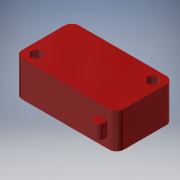
# Autodesk Inventor part: microswitch
Saved by Autodesk Inventor 2019 (Build 230136000, 136)
## iProperties
Created: 2021-01-21
Part Number: microswitch
Material: PET Plastic
Document SubType Name: Modeling
Designer: Juan M. Casillas
Density: 1.541 g/cm^3
Appearance: Smooth - Red
Author: Juan M. Casillas
Autodesk Inventor part; units mm, degrees
ref_plane "YZ Plane" through (0, 0, 0) normal (1, 0, 0) x (0, 1, 0)
ref_plane "XZ Plane" through (0, 0, 0) normal (0, 1, 0) x (-1, 0, 0)
ref_plane "XY Plane" through (0, 0, 0) normal (0, 0, 1) x (1, 0, 0)
sketch "Sketch1" plane through (0, 0, 0) normal (0, 1, 0) x (-1, 0, 0)
  line L0 (12, 7.85) -> (-12, 7.85)
  line L1 (-14, 5.85) -> (-14, -5.85)
  line L2 (-12, -7.85) -> (12, -7.85)
  line L3 (14, -5.85) -> (14, 5.85)
  line L4 (14, 7.85) -> (-14, -7.85) construction
  line L5 (-14, 7.85) -> (14, -7.85) construction
  arc A0 (14, 5.85) -> (12, 7.85) centre (12, 5.85) ccw
  arc A1 (12, -7.85) -> (14, -5.85) centre (12, -5.85) ccw
  arc A2 (-14, -5.85) -> (-12, -7.85) centre (-12, -5.85) ccw
  arc A3 (-12, 7.85) -> (-14, 5.85) centre (-12, 5.85) ccw
  line L6 (12.5, 8.7909) -> (12.5, -11.3064) construction
  line L7 (15.2914, 6.35) -> (1.3637, 6.35) construction
  circle A4 centre (11, 4.85) radius 1.5
  line L8 (14, 0) -> (-14, 0) construction
  line L9 (0, 7.85) -> (0, -7.85) construction
  circle A5 centre (-11.135, -4.985) radius 1.5
  point P0 (0, 0)
  dimension "d0" = 28
  dimension "d1" = 15.7
  dimension "d2" = 2
  dimension "d3" = 1.5
  dimension "d4" = 1.5
  dimension "d5" = 3
  dimension "d15" = 3
  constraints: 20 end point, 10 tangent, 8 point on circle, 8 point on line, 6 centre point, 6 midpoint, 3 equal radius, 2 horizontal, 2 parallel, 1 perpendicular, 1 vertical
  measures "d0" distance of L5.end L4.end
  measures "d1" distance of L4.end L5.start
  measures "d2" radius of A0
  measures "d3" distance between parallel lines of L3 L6
  measures "d4" distance between parallel lines of L0 L7
  measures "d5" diameter of A4
  measures "d15" diameter of A5
extrude "Extrusion1" add sketch "Sketch1" along normal blind 9.7
sketch "Sketch2" plane through (-12, 0, 7.85) normal (0, 0, 1) x (1, 0, 0)
  line L0 (0, 0) -> (24, 0) construction
  line L1 (24, 0) -> (24, 9.7) construction
  line L2 (0, 9.7) -> (24, 9.7) construction
  line L3 (0, 0) -> (0, 9.7) construction
  line L4 (0, 6.7) -> (24, 6.7) construction
  line L5 (24, 0) -> (24, 9.7) construction
  line L6 (0, 9.7) -> (24, 9.7) construction
  line L7 (23.5, 9.7) -> (23.5, 0) construction
  line L8 (0, 0) -> (24, 0) construction
  line L9 (26, 0) -> (26, 9.7) construction
  line L10 (23.5, 6.7) -> (20.7, 6.7)
  line L11 (20.7, 6.7) -> (20.7, 2.8)
  line L12 (20.7, 2.8) -> (23.5, 2.8)
  line L13 (23.5, 2.8) -> (23.5, 6.7)
  point P0 (12, 0)
  dimension "d8" = 3
  dimension "d9" = 2.5
  dimension "d10" = 2.8
  dimension "d11" = 3.9
  constraints: 12 end point, 6 point on line, 3 perpendicular, 2 parallel, 1 horizontal
  measures "d8" distance between parallel lines of L2 L4
  measures "d9" distance between parallel lines of L7 L9
  measures "d10" distance of L12.end L11.end
  measures "d11" distance of L11.end L10.end
extrude "Extrusion2" add sketch "Sketch2" along normal blind 2.3
fillet "Fillet1" radius 1 2 edges at (8.7, 4.75, 10.15) (11.5, 4.75, 10.15)
body "Solid1"
